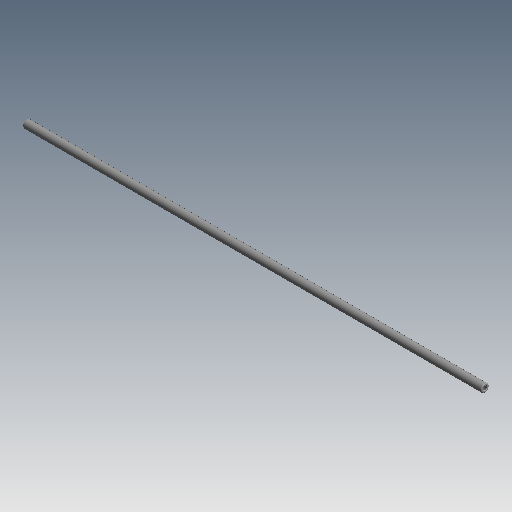
# Autodesk Inventor part: PSSFGW10-582-M6-N6
Saved by Autodesk Inventor 2020 (Build 240168000, 168)
## iProperties
Part Number: PSSFGW10-582-M6-N6
Material: 一般
Catalog Web Link: www.cadenas.de
Description: SFJW, SSFJW, PSFJW, PSSFJW, RSFJW, SFUW, SSFUW, PSFUW, PSSFUW, PSFGW, PSSFGW, SSFGW-Shafts - Both Ends Tapped
Vendor: MISUMI
Document SubType Name: Modeling
Designer: partserver
Manufacturer: MISUMI
Mass: 45.0121 g
Surface Area: 189.621 cm^2
Volume: 45.0121 cm^3
Density: 1 g/cm^3
Appearance: PSOLRGB-175-175-175
Category: PARTsolutions
Company: MISUMI
PSOL_IDENT_0: {$CADENAS_DATA\23d-libs\misumi\metric\01_linear_shafts\rsfjw.prj},479 {VTYP=3D},{NB=PSSFGW10-582-M6-
PSOL_IDENT_1: N6},{LINA=PSSFGW10-582-M6-N6},{NN=SFJW, SSFJW, PSFJW, PSSFJW, RSFJW, SFUW, SSFUW, PSFUW, PSSFUW, PSF
PSOL_IDENT_2: GW, PSSFGW, SSFGW},{DATE=10.11.2021 05:28:16},{GEOMDATE=10.11.2021 05:12:21},{VERSION=},{LINEID=80},
PSOL_IDENT_3: {WBVAR=DTS,MAT,ST,ALT1,L,ALT13,MSC,M,ALT14,NSC,N,ALT3,SC,WSC,X,ALT4,FC,WFC,A,E,ALT7,WKC,CALT7,KC,G,A
PSOL_IDENT_4: LT5,RC,WRC,Y,ALT18,ALT19,ALT40,FCJ,WFCJ,AJ,EJ,HHALT40},{WBNUMERIC=L,MSC,M,NSC,N,SC,WSC,X,FC,WFC,A,E,
PSOL_IDENT_5: WKC,CALT7,KC,G,RC,WRC,Y,FCJ,WFCJ,AJ,EJ,HHALT40}  {NB=PSSFGW10-582-M6-N6},{LINA=PSSFGW10-582-M6-N6},{
PSOL_IDENT_6: KT=DUMMY},{PN=PSSFGW10-582-M6-N6},{TYPE=PSSFGW},{DTS=f8},{DTSALG= 'g6','g6','h5','h5','f8','f8' },{M
PSOL_IDENT_7: AT=SUS304},{MATALG= 'S45C','S45C Equivalent','SUS304','304 Stainless Steel','SUS303','303 Stainless
PSOL_IDENT_8: Steel'  },{ST=HCP10},{STALG= 'HCP10','Hard Chrome Plating - Plating Hardness: HV750~ Plating Thickne
PSOL_IDENT_9: ss: 10 micron or More' },{D=10},{ALT1=},{ALT1ALG= '','w/o LKC (L Dimension Tolerance Change)','LKC','
PSOL_IDENT_10: with LKC (L Dimension Tolerance Change)' },{ALT1PN=},{L=582.0},{LALG=[20:1200/1]},{LMIN=20},{LMAX=12
PSOL_IDENT_11: 00},{ALT13=},{ALT13ALG= '','Not applicable' },{MSC=0},{MSCALG=0},{MSCMIN=0},{MSCMAX=0},{MSCMAX1=228.
PSOL_IDENT_12: 8},{MSCMAX2=0},{MSCMAX3=18},{M=6.0},{MALG=3,4,5,6},{MMIN=3},{MMAX=6},{MMAX1=6},{MMAX2=228.8},{MMAX3=
PSOL_IDENT_13: 30},{MPN=-M6},{ML=12},{UM=19},{PITCH=1},{MPITCH=1},{MSCPITCH=1.5},{ALT14=},{ALT14ALG= '','Not applic
PSOL_IDENT_14: able' },{NSC=0},{NSCALG=0},{NSCALG1=0},{NSCALG2=0},{N=6.0},{NALG=3,4,5,6},{NALG1=3,4,5,6},{NALG2=0},
PSOL_IDENT_15: {NMIN=3},{NPN=-N6},{NL=12},{UN=19},{NPITCH=1},{NSCPITCH=1.5},{CIFMN=0},{CIFPITCH=1},{C=0.5},{ALT3=},
PSOL_IDENT_16: {ALT3ALG= '','w/o Wrench Flats','SC','with SC (Wrench Flats at One Location)','WSC','with WSC (Wrenc
PSOL_IDENT_17: h Flats at Two Locations)' },{ALT3PN=},{SC=0},{SCALG=[0]},{SCMAX=574},{WSC=0},{WSCALG=[0]},{WSCMAX=5
PSOL_IDENT_18: 64},{X=0},{XALG=[0]},{XMAX=564},{W=0},{LL1=0},{LL1ALG=8},{CIFSC=0},{CIFWSC=0},{CIFX=0},{ALT4=},{ALT4
PSOL_IDENT_19: ALG= '','w/o Set Screw Flat','FC','with FC (Set Screw Flat at One Location)','WFC','with WFC (Set Sc
PSOL_IDENT_20: rew Flats at Two Locations)' },{ALT4PN=},{FC=0},{FCALG=[0]},{FCMAX=50},{WFC=0},{WFCALG=[0]},{WFCMAX=
PSOL_IDENT_21: 50},{FC3D=0},{A=0},{AALG=[0]},{AMAX=0},{E=0},{EALG=[0]},{EMAX=580},{HHALT4=0.0},{CIFE=0},{CIFA=0},{A
PSOL_IDENT_22: LT7=},{ALT7ALG= '','Not applicable' },{ALT7PN=},{WKC=0},{WKCALG=[0]},{WKCMAX=580},{CALT7=0},{CALT7AL
PSOL_IDENT_23: G=[0]},{CALT7MIN=0},{CALT7MAX=30},{KC=0},{KCALG=[0]},{KCMAX1=580},{KCMAX2=582},{KCMAX3=580},{G=0},{G
PSOL_IDENT_24: ALG=[0]},{GMIN=0},{GMAX1=30},{GMAX2=30},{GMAX3=30},{BB=0},{BBALG=0},{TT=0.0},{CIFKC=0},{CIFWKC=0},{A
PSOL_IDENT_25: LT5=},{ALT5ALG= '','w/o 90-deg. Set Screw Flat','RC','with RC (90-deg. Set Screw Flat at One Locatio
PSOL_IDENT_26: n)','WRC','with WRC (90-deg. Set Screw Flats at Two Locations)' },{ALT5PN=},{RC=0},{RCALG=[0]},{RCMI
PSOL_IDENT_27: N=2},{RCMAX=582},{WRC=0},{WRCALG=[0]},{WRCMIN=2},{WRCMAX=578},{RC3D=0},{Y=0},{YALG=[0]},{YMIN=2},{YM
PSOL_IDENT_28: AX=580},{BB1=0},{BB1ALG=6},{HHALT5=0.0},{CIFRC=0},{CIFY=0},{ALT18=},{ALT18ALG= '','w/o MD (Left End
PSOL_IDENT_29: Change The Effective Tap Depth to x3)','MD','with MD (Left End Change The Effective Tap Depth to x3)'
PSOL_IDENT_30: },{ALT19=},{ALT19ALG= '','w/o ND (Right End Change The Effective Tap Depth to x3)','ND','with ND (R
PSOL_IDENT_31: ight End Change The Effective Tap Depth to x3)' },{ALT40=},{ALT40ALG= '','w/o Set Screw Flat','FCJ','
PSOL_IDENT_32: with FCJ (Set Screw Flat at One Location)','WFCJ','with WFCJ (Set Screw Flats at Two Locations)' },{
PSOL_IDENT_33: FCJ=0},{FCJALG=[0]},{FCJMAX=50},{WFCJ=0},{WFCJALG=[0]},{WFCJMAX=50},{FCJ3D=0},{AJ=0},{AJALG=[0]},{AJ
PSOL_IDENT_34: MAX=0},{EJ=0},{EJALG=[0]},{EJMAX=580.000},{HHALT40=0},{HHALT40ALG=0},{CIFAJ=0},{CIFEJ=0},{ERRORPN=},
PSOL_IDENT_35: {ERRORMALT3=OK},{ERRORMALT4=OK},{ERRORMALT5=OK},{ERRORMALT7=OK},{ERRORNALT3=OK},{ERRORNALT4=OK},{ERR
PSOL_IDENT_36: ORNALT5=OK},{ERRORNALT7=OK},{ERRORALT34=OK},{ERRORALT35=OK},{ERRORALT37=OK},{ERRORALT45=OK},{ERRORAL
PSOL_IDENT_37: T47=OK},{ERRORALT57=OK},{ERRORMALT40=OK},{ERRORNALT40=OK},{ERRORALT405=OK},{ERRORALT407=OK},{ALT40PN=
PSOL_IDENT_38: }
NB: PSSFGW10-582-M6-N6
NN: SFJW, SSFJW, PSFJW, PSSFJW, RSFJW, SFUW, SSFUW, PSFUW, PSSFUW, PSFGW, PSSFGW, SSFGW
NT: Shafts - Both Ends Tapped
NBSYN: $PN.
LINA: PSSFGW10-582-M6-N6
CATALOG: Misumi
PN: PSSFGW10-582-M6-N6
DTS: f8
MAT: 304 Stainless Steel
ST: Hard Chrome Plating - Plating Hardness: HV750~ Plating Thickness: 10 micron or More
D: 10
ALT1: w/o LKC (L Dimension Tolerance Change)
L: 582
ALT13: Not applicable
MSC: 0
M: 6
ALT14: Not applicable
NSC: 0
N: 6
C: 0.5
ALT3: w/o Wrench Flats
SC: 0
WSC: 0
X: 0
W: 0
LL1: 0
ALT4: w/o Set Screw Flat
FC: 0
WFC: 0
A: 0
E: 0
HHALT4: 0
ALT7: Not applicable
WKC: 0
CALT7: 0
KC: 0
G: 0
BB: 0
TT: 0
ALT5: w/o 90-deg. Set Screw Flat
RC: 0
WRC: 0
Y: 0
BB1: 0
HHALT5: 0
ALT18: w/o MD (Left End Change The Effective Tap Depth to x3)
ALT19: w/o ND (Right End Change The Effective Tap Depth to x3)
SUPPLIER: MISUMI
ARTICLENO: PSSFGW10-582-M6-N6
BOMINFO: PSSFGW10-582-M6-N6
CREATOR: CADENAS GmbH
Title: PSSFGW10-582-M6-N6
Author: Cadenas PARTsolutions
Comments: Shafts - Both Ends Tapped
Autodesk Inventor part; units mm, degrees
ref_plane "YZ Plane" through (0, 0, 0) normal (1, 0, 0) x (0, 1, 0)
ref_plane "XZ Plane" through (0, 0, 0) normal (0, 1, 0) x (-1, 0, 0)
ref_plane "XY Plane" through (0, 0, 0) normal (0, 0, 1) x (1, 0, 0)
sketch "Sketch_1" plane through (0, 0, 0) normal (0, 0, 1) x (1, 0, 0)
  line L0 (582, 0) -> (0, 0)
  line L1 (0, 0) -> (0, 4.5)
  line L2 (0, 4.5) -> (0.5, 5)
  line L3 (0.5, 5) -> (581.5, 5)
  line L4 (581.5, 5) -> (582, 4.5)
  line L5 (582, 4.5) -> (582, 0)
  line L6 (582, 0) -> (0, 0)
  constraints: 14 end point
revolve "Revolution1" add sketch "Sketch_1" angle 360 about axis through (582, 0, 0) along (1, 0, 0)
sketch "Sketch2" plane through (0, 0, 0) normal (-1, 0, 0) x (0, 0, 1)
  point P0 (0, 0)
hole "Hole1" at (0, 0, 0) direction (1, 0, 0) diameter 4.917 depth 17.5806 tip angle 120 countersink diameter 6 countersink angle 90 thread size "M6x1" class "6H" standard "ISO Metric profile"
sketch "Sketch3" plane through (582, 0, 0) normal (1, 0, 0) x (0, 0, -1)
  point P0 (0, 0)
hole "Hole2" at (582, 0, 0) direction (-1, 0, 0) diameter 4.917 depth 17.5806 tip angle 120 countersink diameter 6 countersink angle 90 thread size "M6x1" class "6H" standard "ISO Metric profile"
body "Solid1"
